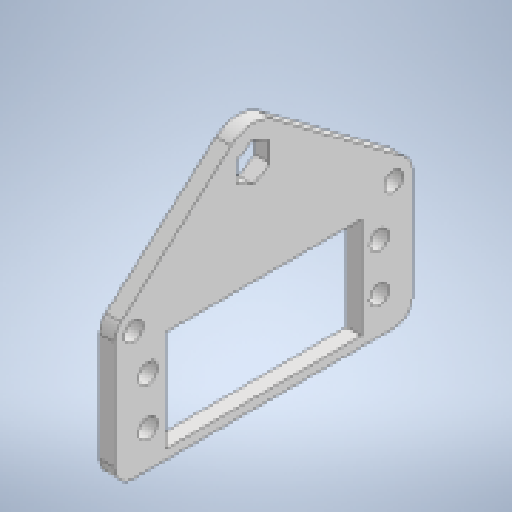
# Autodesk Inventor part: servoPlate
Saved by Autodesk Inventor 2023 (Build 270158000, 158)
## iProperties
Created: 2022-09-10
Part Number: servoPlate
Material: Generic
Document SubType Name: Modeling
Designer: deli
Density: 1 g/cm^3
Appearance: Default
Author: deli
Autodesk Inventor part; units mm, degrees
ref_plane "YZ Plane" through (0, 0, 0) normal (1, 0, 0) x (0, 1, 0)
ref_plane "XZ Plane" through (0, 0, 0) normal (0, 1, 0) x (-1, 0, 0)
ref_plane "XY Plane" through (0, 0, 0) normal (0, 0, 1) x (1, 0, 0)
sketch "Sketch1" plane through (0, 0, 0) normal (1, 0, 0) x (0, 1, 0)
  circle A0 centre (108.0052, 245.4832) radius 2
  circle A1 centre (108.0052, 197.4832) radius 2
  circle A2 centre (98.1052, 197.4832) radius 2
  circle A3 centre (98.1052, 245.4832) radius 2
  line L0 (108.0052, 245.4832) -> (108.0052, 197.4832) construction
  line L1 (108.0052, 197.4832) -> (98.1052, 197.4832) construction
  line L2 (98.1052, 197.4832) -> (98.1052, 245.4832) construction
  line L3 (98.1052, 245.4832) -> (108.0052, 245.4832) construction
  line L4 (113.0552, 248.6332) -> (93.0552, 248.6332) construction
  line L5 (93.0552, 248.6332) -> (93.0552, 194.3332) construction
  line L6 (93.0552, 194.3332) -> (113.0552, 194.3332) construction
  line L7 (113.0552, 194.3332) -> (113.0552, 248.6332) construction
  line L8 (113.0552, 241.3332) -> (93.0552, 241.3332) construction
  line L9 (93.0552, 241.3332) -> (93.0552, 201.6332) construction
  line L10 (93.0552, 201.6332) -> (113.0552, 201.6332) construction
  line L11 (113.0552, 201.6332) -> (113.0552, 241.3332) construction
  line L12 (92.5552, 241.8332) -> (113.5552, 241.8332)
  line L13 (113.5552, 241.8332) -> (113.5552, 201.1332)
  line L14 (113.5552, 201.1332) -> (92.5552, 201.1332)
  line L15 (92.5552, 201.1332) -> (92.5552, 241.8332)
  circle A4 centre (117.0552, 248.4832) radius 2
  circle A5 centre (117.0552, 194.4832) radius 2
  arc A6 (120.041, 251.145) -> (117.0552, 252.4832) centre (117.0552, 248.4832) ccw
  arc A7 (117.0552, 190.4832) -> (120.2678, 192.1001) centre (117.0552, 194.4832) ccw
  arc A8 (90.5552, 194.4832) -> (94.5552, 190.4832) centre (94.5552, 194.4832) ccw
  arc A9 (94.5552, 252.4832) -> (90.5552, 248.4832) centre (94.5552, 248.4832) ccw
  line L16 (121.0552, 248.1479) -> (121.0552, 194.1479) construction
  line L17 (117.0552, 190.4832) -> (94.5552, 190.4832)
  line L18 (90.5552, 194.4832) -> (90.5552, 248.4832)
  line L19 (94.5552, 252.4832) -> (117.0552, 252.4832)
  line L20 (131.0138, 223.7832) -> (133.0345, 227.2832)
  line L21 (133.0345, 227.2832) -> (137.0759, 227.2832)
  line L22 (137.0759, 227.2832) -> (139.0967, 223.7832)
  line L23 (139.0967, 223.7832) -> (137.0759, 220.2832)
  line L24 (137.0759, 220.2832) -> (133.0345, 220.2832)
  line L25 (133.0345, 220.2832) -> (131.0138, 223.7832)
  circle A10 centre (135.0552, 223.7832) radius 7
  line L26 (120.041, 251.145) -> (140.2804, 228.4413)
  line L27 (140.6772, 219.6127) -> (120.2678, 192.1001)
  point P0 (0, 0)
  dimension "d0" = 4
  dimension "d1" = 4
  dimension "d2" = 4
  dimension "d3" = 4
  dimension "d4" = 9.9
  dimension "d5" = 48
  dimension "d7" = 20
  dimension "d8" = 5.05
  dimension "d9" = 3.15
  dimension "d10" = 39.7
  dimension "d11" = 7.3
  dimension "d12" = 0.5
  dimension "d14" = 4
  dimension "d16" = 4
  dimension "d18" = 2
  dimension "d20" = 2
  dimension "d28" = 54
  dimension "d30" = 2
  dimension "d31" = 7.5
  dimension "d32" = 62
  dimension "d33" = 3.85
  dimension "d34" = 54.3
  dimension "d35" = 7
  dimension "d36" = 14
  dimension "d37" = 14
  dimension "d40" = 54
  dimension "d41" = 26.3
  constraints: 56 end point, 12 tangent, 11 centre point, 10 point on circle, 9 perpendicular, 6 parallel, 3 coincident, 3 horizontal, 2 point on line, 2 vertical, 16 other
  measures "d0" diameter of A0
  measures "d1" diameter of A3
  measures "d2" diameter of A1
  measures "d3" diameter of A2
  measures "d4" distance of L2.end L0.start
  measures "d5" distance of L0.start L0.end
  measures "d7" distance of L5.end L6.end
  measures "d8" distance between parallel lines of L0 L7
  measures "d9" distance between parallel lines of L6 L1
  measures "d10" distance of L10.end L8.start
  measures "d11" distance between parallel lines of L6 L10
  measures "d12" distance between parallel lines of L8 L12
  measures "d14" diameter of A4
  measures "d16" diameter of A5
  measures "d18" radial gap between concentric circles of A6 A4
  measures "d20" radial gap between concentric circles of A5 A7
  measures "d28" distance of L16.start L16.end
  measures "d30" distance between parallel lines of L15 L18
  measures "d31" distance between parallel lines of L16 L13
  measures "d32" distance between parallel lines of L17 L19
  measures "d33" distance between parallel lines of L19 L4
  measures "d34" distance of L6.end L4.start
  measures "d35" distance between parallel lines of L24 L21
  measures "d36" diameter of A10
  measures "d37" distance from line of L16 point (135.055, 223.783)
  measures "d40" distance of A5.centre A4.centre
  measures "d41" vertical distance of L0.end A10.centre
extrude "Extrusion2" add sketch "Sketch1" along normal blind 3.175
equation "\"d1\" = d0"
equation "\"d2\" = d0"
equation "\"d3\" = d0"
equation "\"d8\" = -0.5 * d4 + 0.5 * d7"
equation "\"d9\" = -0.5 * d5 + 0.5 * d6"
equation "\"d11\" = -0.5 * d10 + 0.5 * d6"
equation "\"d14\" = d13"
equation "\"d16\" = d13"
equation "\"d18\" = d17"
equation "\"d20\" = d17"
equation "\"d33\" = -0.5 * d34 + 0.5 * d32"
equation "\"d40\" = d28"
equation "\"d6\" = 54.3"
equation "\"d13\" = 4"
equation "\"d17\" = 2"
body "Solid2"
